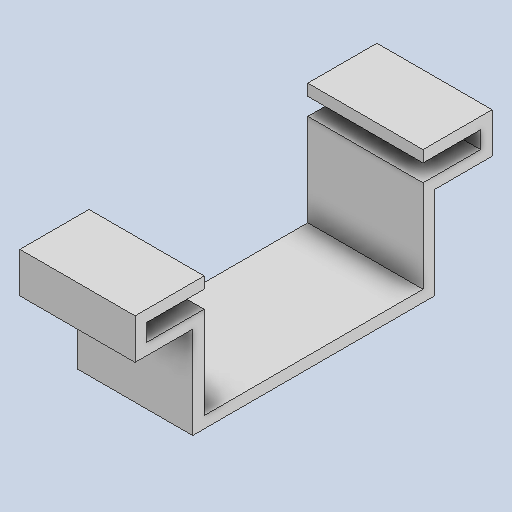
# Autodesk Inventor part: Drziak_1
Saved by Autodesk Inventor 2025 (Build 290162000, 162)
## iProperties
Created: 2025-06-09
Part Number: Drziak_1
Material: Generic
Document SubType Name: Modeling
Designer: Pravoslav
Density: 1 g/cm^3
Appearance: Default
Author: Pravoslav
Autodesk Inventor part; units mm, degrees
ref_plane "YZ Plane" through (0, 0, 0) normal (1, 0, 0) x (0, 1, 0)
ref_plane "XZ Plane" through (0, 0, 0) normal (0, 1, 0) x (-1, 0, 0)
ref_plane "XY Plane" through (0, 0, 0) normal (0, 0, 1) x (1, 0, 0)
sketch "Sketch1" plane through (0, 0, 0) normal (1, 0, 0) x (0, 1, 0)
  line L0 (0, 9.5) -> (0, -9.5)
  line L1 (0, -9.5) -> (8, -9.5)
  line L2 (0, 9.5) -> (8, 9.5)
  line L3 (8, 9.5) -> (8, 14.5)
  line L4 (8, 14.5) -> (9.5, 14.5)
  line L5 (9.5, 14.5) -> (9.5, 9.5)
  line L6 (9.5, 9.5) -> (10.5, 9.5)
  line L7 (10.5, 9.5) -> (10.5, 15.5)
  line L8 (10.5, 15.5) -> (7, 15.5)
  line L9 (7, 15.5) -> (7, 10.5)
  line L10 (7, 10.5) -> (0, 10.5)
  line L11 (0, 10.5) -> (-1, 10.5)
  line L12 (-1, 10.5) -> (-1, 0)
  line L13 (0, 0) -> (3.5, 0)
  line L14 (0, -9.5) -> (8, -9.5)
  line L15 (8, -9.5) -> (8, -14.5)
  line L16 (8, -14.5) -> (9.5, -14.5)
  line L17 (9.5, -14.5) -> (9.5, -9.5)
  line L18 (10.5, -9.5) -> (10.5, -15.5)
  line L19 (10.5, -15.5) -> (7, -15.5)
  line L20 (7, -15.5) -> (7, -10.5)
  line L21 (7, -10.5) -> (0, -10.5)
  line L22 (0, -10.5) -> (-1, -10.5)
  line L23 (-1, -10.5) -> (-1, 0)
  line L24 (10.5, -9.5) -> (9.5, -9.5)
  dimension "d0" = 19
  dimension "d1" = 0
  dimension "d2" = 8
  dimension "d3" = 8
  dimension "d4" = 5
  dimension "d5" = 1.5
  dimension "d6" = 1
  dimension "d7" = 6
  dimension "d8" = 3.5
  dimension "d9" = 5
  dimension "d10" = 1
  constraints: 50 end point, 9 symmetric about line, 8 perpendicular, 4 horizontal, 2 point on line, 2 vertical, 1 midpoint
  measures "d0" distance of L0.start L0.end
  measures "d1" distance of point (0, 0) L13.start
  measures "d2" distance of L0.end L1.end
  measures "d3" distance of L0.start L2.end
  measures "d4" distance of L2.end L3.end
  measures "d5" distance of L3.end L4.end
  measures "d6" distance of L5.end L6.end
  measures "d7" distance of L6.end L7.end
  measures "d8" distance of L7.end L8.end
  measures "d9" distance of L8.end L9.end
  measures "d10" distance of L10.end L11.end
extrude "Extrusion1" add sketch "Sketch1" along normal blind 10
body "Solid1"
